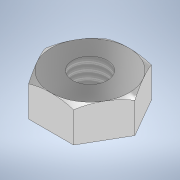
# Autodesk Inventor part: M3-HexaNut-type2
Saved by Autodesk Inventor 2022.2 (Build 262287000, 287)
## iProperties
Created: 2022-02-28
Part Number: M3-HexaNut-type2
Material: 一般
Document SubType Name: Modeling
Designer: Yuta Fujiyama
Density: 1 g/cm^3
Appearance: クローム - つや出し
Author: Yuta Fujiyama
Autodesk Inventor part; units mm, degrees
ref_plane "YZ Plane" through (0, 0, 0) normal (1, 0, 0) x (0, 1, 0)
ref_plane "XZ Plane" through (0, 0, 0) normal (0, 1, 0) x (-1, 0, 0)
ref_plane "XY Plane" through (0, 0, 0) normal (0, 0, 1) x (1, 0, 0)
sketch "スケッチ1" plane through (0, 0, 0) normal (0, 1, 0) x (-1, 0, 0)
  circle A0 centre (0, 0) radius 3.1754 construction
  line L0 (3.1754, 0) -> (1.5877, 2.75)
  line L1 (1.5877, 2.75) -> (-1.5877, 2.75)
  line L2 (-1.5877, 2.75) -> (-3.1754, 0)
  line L3 (-3.1754, 0) -> (-1.5877, -2.75)
  line L4 (-1.5877, -2.75) -> (1.5877, -2.75)
  line L5 (1.5877, -2.75) -> (3.1754, 0)
  dimension "d0" = 5.5
  constraints: 12 end point, 6 point on circle, 4 equal length, 2 horizontal, 1 centre point, 1 coincident
  measures "d0" distance between parallel lines of L4 L1
extrude "押し出し1" add sketch "スケッチ1" along normal blind 2.4
sketch "スケッチ2" plane through (0, 2.4, 0) normal (0, 1, 0) x (1, 0, 0)
  point P0 (0, 0)
  point P1 (0, 0)
  constraints: 1 coincident
hole "穴1" at (0, 2.4, 0) direction (0, -1, 0) diameter 2.459 end through all thread size "M3x0.5" class "6H" standard "ISO Metric profile"
sketch "スケッチ3" plane through (0, 0, 0) normal (1, 0, 0) x (0, 1, 0)
  arc A0 (1.7511, -3.75) -> (2.4, -2.75) centre (-2.9327, 0) ccw
  line L0 (0, -2.75) -> (2.4, -2.75) construction
  line L1 (2.4, -3.75) -> (1.7511, -3.75)
  line L2 (2.4, 1.2295) -> (2.4, -1.2295) construction
  line L3 (2.4, -2.75) -> (2.4, -3.75)
  line L4 (-4.0042, 0) -> (3.4964, 0) projected
  point P0 (0, 0)
  point P1 (2.4, 0)
  dimension "d10" = 2.75
  dimension "d11" = 6
  dimension "d12" = 1
  constraints: 4 end point, 2 point on circle, 1 centre point, 1 collinear, 1 horizontal alignment, 1 midpoint, 1 perpendicular
  measures "d10" distance of L3.start point (2.4, 0)
  measures "d11" radius of A0
  measures "d12" distance of L3.start L1.start
revolve "回転1" cut sketch "スケッチ3" angle 360 about axis through (0, -10, 0) along (0, 1, 0)
